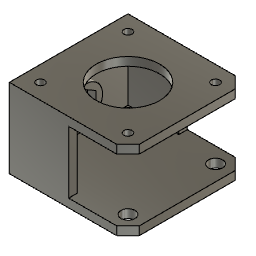
belt_tensioner (Autodesk Fusion 360 design; units mm, degrees)
Autodesk Fusion 360 part; units mm, degrees
sketch "Sketch1" plane through (0, 0, 0) normal (0, 0, 1) x (1, 0, 0)
  line L0 (21, 21) -> (-21, 21)
  line L1 (-21, 21) -> (-21, -21)
  line L2 (-21, -21) -> (21, -21)
  line L3 (21, -21) -> (21, 21)
  line L4 (21, 21) -> (-21, -21) construction
  line L5 (-21, 21) -> (21, -21) construction
  circle A0 centre (0, 0) radius 11.2
  circle A1 centre (15.5, 15.5) radius 1.45
  circle A2 centre (-15.5, 15.5) radius 1.45
  circle A3 centre (-15.5, -15.5) radius 1.45
  circle A4 centre (15.5, -15.5) radius 1.45
  line L6 (-18, 18) -> (18, 18)
  line L7 (18, 18) -> (18, -18)
  line L8 (18, -18) -> (-18, -18)
  line L9 (-18, -18) -> (-18, 18)
  line L10 (-18, 18) -> (18, -18) construction
  line L11 (18, 18) -> (-18, -18) construction
  line L12 (21, 21) -> (21, 18)
  line L13 (21, -21) -> (21, -18)
  line L14 (0, -18) -> (0, -21)
  line L15 (0, 21) -> (0, 18)
  line L16 (-205.75, 0) -> (209.25, 0)
  dimension "d43" = 42
  dimension "d44" = 22.4
  dimension "d45" = 2.9
  dimension "d46" = 31
  dimension "d60" = 3
  constraint horizontal L0
  constraint perpendicular L0 L1
  constraint parallel L0 L2
  constraint parallel L1 L3
  constraint coincident L4 A0.centre
  constraint coincident L5 A0.centre
  constraint coincident A0.centre origin
  constraint equal L0 L3
  constraint coincident L4 A1.centre
  constraint coincident L5 A2.centre
  constraint coincident L4 A3.centre
  constraint coincident L5 A4.centre
  constraint horizontal A1.centre A2.centre
  constraint vertical A1.centre A4.centre
  constraint horizontal A3.centre A4.centre
  constraint equal A1 A4
  constraint equal A3 A4
  constraint equal A2 A3
  constraint horizontal L6
  constraint perpendicular L6 L7
  constraint parallel L6 L8
  constraint parallel L7 L9
  constraint coincident L10 A0.centre
  constraint coincident L11 A0.centre
  constraint equal L6 L9
  constraint coincident L6 L12.end
  constraint perpendicular L6 L12
  constraint coincident L8 L13.end
  constraint perpendicular L8 L13
  constraint midpoint L8 L14.start
  constraint midpoint L2 L14.end
  constraint midpoint L0 L15.start
  constraint midpoint L6 L15.end
  measures "d43" distance of L0.start L2.end
  measures "d44" diameter of A0
  measures "d45" diameter of A1
  measures "d46" distance of A1.centre A2.centre
  measures "d60" distance of L1 L9
extrude "Extrude1" add sketch "Sketch1" along normal blind 3 contours L0 L3 L6 L7 L12 L15 L16 | L0 L1 L6 L9 L15 L16 | A0 L6 L7 L9 L16 | L2 L3 L7 L8 L13 L14 L16 | L1 L2 L8 L9 L14 L16 | A0 L7 L8 L9 L16
extrude "Extrude2" add sketch "Sketch1" against normal blind 25 contours L0 L1 L6 L9 L15 L16 | L1 L2 L8 L9 L14 L16
extrude "Extrude3" add sketch "Sketch1" along normal blind 3 from surface at -25 contours L0 L3 L6 L7 L12 L15 L16 | L0 L1 L6 L9 L15 L16 | A0 L6 L7 L9 L16 | L2 L3 L7 L8 L13 L14 L16 | L1 L2 L8 L9 L14 L16 | A0 L7 L8 L9 L16 | A0 L16 | A0 L16 | A1 | A2 | A3 | A4
sketch "Sketch2" plane through (0, 0, -25) normal (0, 0, -1) x (1, 0, 0)
  line L0 (21, -21) -> (21, 21)
  line L1 (21, 21) -> (-21, 21)
  line L2 (-21, 21) -> (-21, -21)
  line L3 (-21, -21) -> (21, -21)
  circle A0 centre (0, 0) radius 2
  dimension "d62" = 4
  constraint coincident A0.centre origin
  measures "d62" diameter of A0
sketch "Sketch4" plane through (-18, 0, 0) normal (1, 0, 0) x (0, 1, 0)
  circle A0 centre (0, -11) radius 2.2
  line L0 (0, -11) -> (-18, -11) construction
  line L1 (0, -6.7276) -> (-3.7, -8.8638)
  line L2 (-3.7, -8.8638) -> (-3.7, -13.1362)
  line L3 (-3.7, -13.1362) -> (0, -15.2724)
  line L4 (0, -15.2724) -> (3.7, -13.1362)
  line L5 (3.7, -13.1362) -> (3.7, -8.8638)
  line L6 (3.7, -8.8638) -> (0, -6.7276)
  circle A1 centre (0, -11) radius 6
  line L7 (-18, -22) -> (18, -22)
  line L8 (18, -22) -> (18, 0)
  line L9 (18, 0) -> (-18, 0)
  line L10 (-18, 0) -> (-18, -22)
  point P0 (0, -11)
  dimension "d1" = 4.4
  dimension "d2" = 7.4
  dimension "d3" = 12
  constraint coincident P0 A0.centre
  constraint horizontal L0
  constraint vertical L5
  constraint midpoint L0.end L10
  constraint vertical origin A0.centre
  measures "d1" diameter of A0
  measures "d2" distance of L2 L5
  measures "d3" diameter of A1
extrude "Extrude5" cut sketch "Sketch4" against normal blind 59 contours A0
extrude "Extrude10" add sketch "Sketch4" along normal blind 3 contours A1
sketch "Sketch3" plane through (0, 0, -22) normal (0, 0, 1) x (-1, 0, 0)
  line L0 (0, -18) -> (18, -18)
  line L1 (18, -18) -> (18, 18)
  line L2 (18, 18) -> (0, 18)
  circle A0 centre (-15.5, 15.5) radius 1.45
  circle A1 centre (15.5, 15.5) radius 1.45
  circle A2 centre (15.5, -15.5) radius 1.45
  circle A3 centre (-15.5, -15.5) radius 1.45
  circle A4 centre (-15.5, 15.5) radius 2.5
  circle A5 centre (15.5, 15.5) radius 2.5
  circle A6 centre (15.5, -15.5) radius 2.5
  circle A7 centre (-15.5, -15.5) radius 2.5
  line L3 (0, 18) -> (0, 21)
  line L4 (0, 21) -> (-21, 21)
  line L5 (-21, 21) -> (-21, -21)
  line L6 (-21, -21) -> (0, -21)
  line L7 (0, -21) -> (0, -18)
  dimension "d104" = 5
  dimension "d105" = 5
  constraint concentric A0 A4
  constraint concentric A1 A5
  constraint tangent L2 A5
  constraint concentric A2 A6
  constraint tangent L1 A6
  constraint concentric A3 A7
  measures "d104" diameter of A4
  measures "d105" diameter of A7
extrude "Extrude11" cut sketch "Sketch3" against normal blind 5 contours A6 | A5 | A0 | A1 | A2 | A3 | A4 | A7
chamfer "Chamfer1" distance 4 angle 45 4 edges at (21, 21, 1.5) (21, -21, 1.5) (21, 21, -23.5) (21, -21, -23.5)
equation "d44 = 22 mm + x2gap"
equation "d45 = 2.5 mm + x2gap"
equation "x2gap = 0.4 mm"
equation "d1 = 4 mm + x2gap"
equation "d2 = 7 mm + x2gap"
